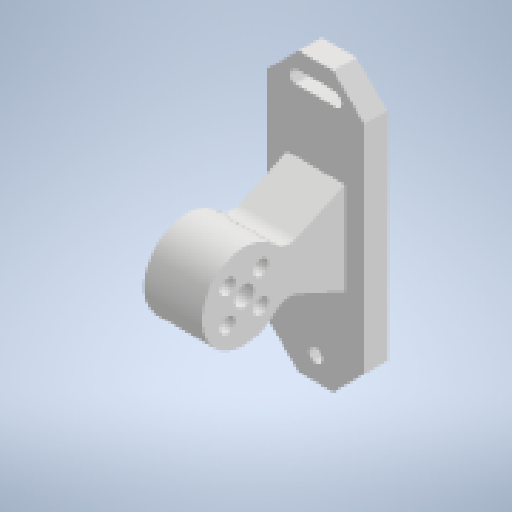
# Autodesk Inventor part: FiberCoupler
Saved by Autodesk Inventor 2023.1 (Build 271208000, 208)
## iProperties
Created: 2023-06-07
Part Number: FiberCoupler
Material: Generic
Document SubType Name: Modeling
Designer: hello
Density: 1 g/cm^3
Appearance: Default
Author: hello
Autodesk Inventor part; units mm, degrees
ref_plane "YZ Plane" through (0, 0, 0) normal (1, 0, 0) x (0, 1, 0)
ref_plane "XZ Plane" through (0, 0, 0) normal (0, 1, 0) x (-1, 0, 0)
ref_plane "XY Plane" through (0, 0, 0) normal (0, 0, 1) x (1, 0, 0)
sketch "Sketch1" plane through (0, 0, 0) normal (1, 0, 0) x (0, 1, 0)
  line L0 (-36, 0) -> (36, 0)
  line L1 (36, 0) -> (36, 6)
  line L2 (36, 6) -> (-36, 6)
  line L3 (-36, 6) -> (-36, 0)
  circle A0 centre (0, 32) radius 9
  circle A1 centre (0, 32) radius 11
  line L4 (0, 32) -> (3.7715, 23.8284) construction
  line L5 (4.6096, 22.0124) -> (12, 6)
  line L6 (0, 32) -> (-3.7715, 23.8284) construction
  line L7 (-4.6096, 22.0124) -> (-12, 6)
  line L8 (11, 32) -> (9, 32)
  line L9 (-9, 32) -> (-11, 32)
  point P0 (0, 0)
  point P1 (0, 0)
  point P2 (10, 32)
  dimension "d3" = 18
  dimension "d4" = 32
  dimension "d5" = 6
  dimension "d6" = 72
  dimension "d7" = 2
  dimension "d44" = 12
  dimension "d45" = 12
  constraints: 20 end point, 8 point on circle, 4 point on line, 2 centre point, 2 collinear, 2 horizontal, 2 midpoint, 2 parallel, 1 coincident, 1 horizontal alignment, 1 perpendicular, 1 vertical alignment
  measures "d3" diameter of A0
  measures "d4" distance of point (0, 0) L4.start
  measures "d5" distance of L0.end L1.end
  measures "d6" distance of L0.start L0.end
  measures "d7" radial gap between concentric circles of A0 A1
  measures "d44" horizontal distance of L7.end point (0, 0)
  measures "d45" horizontal distance of L5.end point (0, 0)
extrude "Extrusion1" add sketch "Sketch1" along normal mid plane 7
sketch "Sketch2" plane through (3.5, 0, 0) normal (1, 0, 0) x (0, 0, -1)
  line L0 (-6, 36) -> (-6, 12) projected
  line L1 (-6, 12) -> (-22.0124, 4.6096) projected
  arc A0 (-22.0124, 4.6096) -> (-22.0124, -4.6096) centre (-32, 0) ccw projected
  line L2 (-22.0124, -4.6096) -> (-6, -12) projected
  line L3 (-6, -12) -> (-6, -36) projected
  line L4 (-6, -36) -> (0, -36) projected
  line L5 (0, -36) -> (0, 36) projected
  line L6 (0, 36) -> (-6, 36) projected
  line L7 (-32, -9) -> (-32, -15) projected
  point P0 (0, 0)
extrude "Extrusion2" add sketch "Sketch2" along normal blind 4
sketch "Sketch3" plane through (-3.5, 0, 0) normal (-1, 0, 0) x (0, 0, 1)
  line L0 (22.0124, -4.6096) -> (6, -12) projected
  line L1 (6, -12) -> (6, -36) projected
  line L2 (6, -36) -> (0, -36) projected
  line L3 (0, -36) -> (0, 36) projected
  line L4 (0, 36) -> (6, 36) projected
  line L5 (6, 36) -> (6, 12) projected
  line L6 (6, 12) -> (22.0124, 4.6096) projected
  arc A0 (22.0124, -4.6096) -> (22.0124, 4.6096) centre (32, 0) ccw projected
  point P0 (0, 0)
extrude "Extrusion3" add sketch "Sketch3" along normal blind 4
sketch "Sketch4" plane through (7.5, -36, 0) normal (0, 0, -1) x (-1, 0, 0)
  line L0 (15, 72) -> (15, 0) projected
  line L1 (0, 0) -> (0, 72) projected
  line L2 (15, 0) -> (20, 0)
  line L3 (20, 0) -> (20, 72)
  line L4 (20, 72) -> (15, 72)
  line L5 (15, 72) -> (15, 0)
  line L6 (0, 0) -> (-5, 0)
  line L7 (-5, 0) -> (-5, 72)
  line L8 (-5, 72) -> (0, 72)
  line L9 (0, 72) -> (0, 0)
  point P0 (7.5, 36)
  dimension "d17" = 25
  constraints: 16 end point, 4 parallel, 2 horizontal, 2 perpendicular, 1 collinear
  measures "d17" distance of L7.end L3.end
extrude "Extrusion4" add sketch "Sketch4" against normal up to surface (6 mm away)
fillet "Fillet1" radius 5 4 edges at (-5.5, 4.6096, 22.0124) (2, 4.6096, 22.0124) (-5.5, -4.6096, 22.0124) (2, -4.6096, 22.0124)
sketch "Sketch10" plane through (-12.5, 36, 6) normal (0, 0, 1) x (1, 0, 0)
  line L0 (12.5, -66) -> (12.5, -6)
  line L1 (0, 0) -> (25, 0) projected
  circle A0 centre (12.5, -66) radius 1.75
  arc A1 (17.5, -6.2087) -> (7.5, -6.2087) centre (12.5, -66) ccw construction
  arc A2 (17.6458, -4.4648) -> (7.3542, -4.4648) centre (12.5, -66) ccw
  arc A3 (17.3542, -7.9526) -> (7.6458, -7.9526) centre (12.5, -66) ccw
  arc A4 (17.3542, -7.9526) -> (17.6458, -4.4648) centre (17.5, -6.2087) ccw
  arc A5 (7.3542, -4.4648) -> (7.6458, -7.9526) centre (7.5, -6.2087) ccw
  point P0 (12.5, -36)
  point P1 (12.5, -36)
  dimension "d46" = 60
  dimension "d47" = 3.5
  dimension "d48" = 3.5
  dimension "d49" = 5
  constraints: 11 point on circle, 6 centre point, 4 tangent, 3 coincident, 2 end point, 1 midpoint, 1 perpendicular
  measures "d46" distance of L0.end L0.start
  measures "d47" diameter of A0
  measures "d48" diameter of A4
  measures "d49" distance from line of A1.end L0
extrude "Extrusion5" cut sketch "Sketch10" against normal through all
chamfer "Chamfer1" distance 8 angle 45 4 edges at (12.5, 36, 3) (-12.5, 36, 3) (12.5, -36, 3) (-12.5, -36, 3)
sketch "Sketch11" plane through (-7.5, 0, 0) normal (-1, 0, 0) x (0, 0, 1)
  arc A0 (23.9532, -7.4999) -> (23.9532, 7.4999) centre (32, 0) ccw projected
  point P0 (0, 0)
  constraints: 1 coincident
hole "Hole3" at (-7.5, 0, 32) direction (1, 0, 0) diameter 5 depth 15 counterbore diameter 16 counterbore depth 9
sketch "Sketch12" plane through (7.5, 0, 0) normal (1, 0, 0) x (0, 0, -1)
  circle A0 centre (-32, 0) radius 2.5 projected
  line L0 (-36.3, -4.3) -> (-27.7, -4.3)
  line L1 (-27.7, -4.3) -> (-27.7, 4.3)
  line L2 (-27.7, 4.3) -> (-36.3, 4.3)
  line L3 (-36.3, 4.3) -> (-36.3, -4.3)
  line L4 (-36.3, -4.3) -> (-27.7, 4.3) construction
  line L5 (-27.7, -4.3) -> (-36.3, 4.3) construction
  point P0 (0, 0)
  dimension "d67" = 8.6
  dimension "d68" = 8.6
  constraints: 12 end point, 4 coincident, 2 midpoint, 2 parallel, 1 horizontal, 1 perpendicular
  measures "d67" distance of L2.end L1.end
  measures "d68" distance of L1.end L0.end
hole "Hole4" at (7.5, -4.3, 36.3) at (7.5, 4.3, 36.3) at (7.5, 4.3, 27.7) at (7.5, -4.3, 27.7) direction (-1, 0, 0) diameter 3.9 depth 5
equation "\"d3\" = LENS_D"
equation "\"d45\" = d44"
equation "\"d10\" = LENS_L"
equation "\"LENS_D\" = 18"
equation "\"LENS_L\" = 7"
equation "\"LENS_R\" = 25"
body "Solid1"
